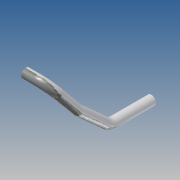
# Autodesk Inventor part: exhaust header right pipe 1
Saved by Autodesk Inventor 2013 (Build 170138000, 138)
## iProperties
Created: 2013-02-09
Part Number: exhaust header right pipe 1
Material: Steel
Document SubType Name: Modeling
Designer: zhaphod
Density: 1 g/cm^3
Author: zhaphod
Autodesk Inventor part; units mm, degrees
sketch "Sketch1" plane through (0, 0, 0) normal (1, 0, 0) x (0, 1, 0)
  line L0 (0, 0) -> (121.2, -150)
  line L1 (121.2, -150) -> (273.35, -287.775)
  line L2 (273.35, -287.775) -> (463.85, -287.775)
  line L3 (0, 0) -> (0, -103.1875) construction
  line L4 (0, -103.1875) -> (121.2, -109.925) construction
  line L5 (121.2, -109.925) -> (273.35, -97.225) construction
  line L6 (273.35, -97.225) -> (463.85, -97.225) construction
  dimension "d0" = 287.775
  dimension "d4" = 150
  dimension "d5" = 463.85
  dimension "d6" = 103.1875
  dimension "d7" = 97.225
  dimension "d8" = 109.925
  dimension "d19" = 121.2
  dimension "d20" = 190.5
  constraints: 14 end point, 3 vertical alignment, 2 perpendicular, 1 horizontal
  measures "d0" distance from line of L2 L0.start
  measures "d4" vertical distance of L0.end L0.start
  measures "d5" horizontal distance of L0.start L2.end
  measures "d6" distance of L0.start L3.end
  measures "d7" distance from line of L6 L0.start
  measures "d8" vertical distance of L4.end L0.start
  measures "d19" horizontal distance of L0.end L0.start
  measures "d20" distance of L1.end L2.end
ref_plane "Work Plane1" through (103.1875, 0, 0) normal (1, 0, 0) x (0, 1, 0)
ref_plane "Work Plane2" through (109.925, 0, 0) normal (1, 0, 0) x (0, 1, 0)
ref_plane "Work Plane3" through (97.225, 0, 0) normal (1, 0, 0) x (0, 1, 0)
sketch "Sketch2" plane through (103.1875, 0, 0) normal (1, 0, 0) x (0, 1, 0)
  point P0 (0, 0)
  point P1 (0, 0)
sketch "Sketch3" plane through (109.925, 0, 0) normal (1, 0, 0) x (0, 1, 0)
  point P0 (0, 0)
  point P1 (121.2, -150)
  point P2 (273.35, -287.775)
sketch "Sketch4" plane through (97.225, 0, 0) normal (1, 0, 0) x (0, 1, 0)
  point P0 (0, 0)
  point P1 (463.85, -287.775)
  point P2 (273.35, -287.775)
sketch "Sketch5" plane through (0, 0, 0) normal (1, 0, 0) x (0, 1, 0)
  circle A0 centre (0, 0) radius 20.6375
  circle A1 centre (0, 0) radius 19.0375
  dimension "d15" = 1.6
  dimension "d17" = 41.275
  constraints: 2 centre point, 2 coincident
  measures "d15" radial gap between concentric circles of A0 A1
  measures "d17" diameter of A0
sketch3d "3D Sketch1"
  line L0 (0, 0, 0) -> (43.4003, 0, 0)
  arc A0 (43.4003, 0, 0) -> (105.275, 37.5523, -46.4756) centre (43.4003, 38.9109, -48.157) ccw
  line L1 (105.275, 37.5523, -46.4756) -> (109.7267, 117.6333, -145.5858)
  arc A1 (109.7267, 117.6333, -145.5858) -> (109.5743, 125.4012, -153.8043) centre (77.0227, 159.232, -113.4431) ccw
  line L2 (109.5743, 125.4012, -153.8043) -> (98.7035, 255.6374, -271.7359)
  arc A2 (98.7035, 255.6374, -271.7359) -> (97.225, 297.291, -287.775) centre (102.908, 297.291, -226.1239) ccw
  line L3 (97.225, 297.291, -287.775) -> (97.225, 463.85, -287.775)
  dimension "d12" = 61.9125
  dimension "d13" = 61.9125
  dimension "d14" = 61.9125
sweep "Sweep1" add profiles "Sketch5" path "3D Sketch1"
equation "\"d13\" = d12"
equation "\"d14\" = d12"
equation "\"d9\" = d6"
equation "\"d10\" = d8"
equation "\"d11\" = d7"
body "Solid1"
